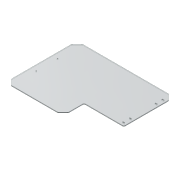
# Autodesk Inventor part: Clear Front Door 2
Saved by Autodesk Inventor 2015 (Build 190159000, 159)
## iProperties
Created: 2018-04-14
Part Number: Clear Front Door 2
Material: Glass
Document SubType Name: Modeling
Designer: Ghassan Yusuf
Density: 2.18 g/cm^3
Appearance: Clear
Author: Ghassan Yusuf
Autodesk Inventor part; units mm, degrees
ref_plane "YZ Plane" through (0, 0, 0) normal (1, 0, 0) x (0, 1, 0)
ref_plane "XZ Plane" through (0, 0, 0) normal (0, 1, 0) x (-1, 0, 0)
ref_plane "XY Plane" through (0, 0, 0) normal (0, 0, 1) x (1, 0, 0)
sketch "TFT LCD Touch Screen" plane through (0, 0, 0) normal (0, 0, 1) x (1, 0, 0)
  line L0 (-55, 32.5) -> (55, 32.5)
  line L1 (55, 32.5) -> (55, -32.5)
  line L2 (55, -32.5) -> (-55, -32.5)
  line L3 (-55, -32.5) -> (-55, 32.5)
  circle A0 centre (-51, 28.5) radius 1.5
  circle A1 centre (-51, -28.5) radius 1.5
  circle A2 centre (51, -28.5) radius 1.5
  circle A3 centre (51, 28.5) radius 1.5
  line L4 (-40, 29) -> (40, 29)
  line L5 (40, 29) -> (40, -29)
  line L6 (40, -29) -> (-40, -29)
  line L7 (-40, -29) -> (-40, 29)
  point P0 (0.75, 3.075)
  point P1 (0, 32.5)
  point P2 (55, 0)
  point P3 (0, 29)
  point P4 (-40, 0)
  dimension "d9" = 110
  dimension "d10" = 65
  dimension "d11" = 3
  dimension "d12" = 57
  dimension "d13" = 102
  dimension "d14" = 4
  dimension "d15" = 4
  dimension "d16" = 80
  dimension "d17" = 58
  measures "d9" distance of L1.end L2.end
  measures "d10" distance of L0.end L1.end
  measures "d11" diameter of A0
  measures "d12" distance of A0.centre A1.centre
  measures "d13" distance of A3.centre A0.centre
  measures "d14" distance from line of L0 A3.centre
  measures "d15" distance from line of L3 A0.centre
  measures "d16" distance of L5.end L6.end
  measures "d17" distance of L4.end L5.end
sketch "Hinges Screw Holes" plane through (0, 0, 0) normal (0, 0, 1) x (1, 0, 0)
  arc A0 (172, 94.429) -> (172, 97.929) centre (172, 96.179) ccw
  arc A1 (172, 68.929) -> (172, 72.429) centre (172, 70.679) ccw
  arc A2 (172, -27.2) -> (172, -23.7) centre (172, -25.45) ccw
  arc A3 (172, -52.7) -> (172, -49.2) centre (172, -50.95) ccw
  arc A4 (167, 97.929) -> (167, 94.429) centre (167, 96.179) ccw
  arc A5 (167, 72.429) -> (167, 68.929) centre (167, 70.679) ccw
  arc A6 (167, -23.7) -> (167, -27.2) centre (167, -25.45) ccw
  arc A7 (167, -49.2) -> (167, -52.7) centre (167, -50.95) ccw
  line L0 (167, 97.929) -> (172, 97.929)
  line L1 (167, 94.429) -> (172, 94.429)
  line L2 (167, 72.429) -> (172, 72.429)
  line L3 (167, 68.929) -> (172, 68.929)
  line L4 (167, -23.7) -> (172, -23.7)
  line L5 (167, -27.2) -> (172, -27.2)
  line L6 (167, -49.2) -> (172, -49.2)
  line L7 (167, -52.7) -> (172, -52.7)
  point P0 (169.5, 0)
  point P1 (0, -7.5)
  dimension "d47" = 3.5
  dimension "d48" = 3.5
  dimension "d50" = 25.5
  dimension "d51" = 3.5
  dimension "d52" = 3.5
  dimension "d53" = 25.5
  dimension "d58" = 3.5
  dimension "d59" = 3.5
  dimension "d60" = 25.5
  dimension "d61" = 3.5
  dimension "d62" = 3.5
  dimension "d63" = 25.5
  dimension "d65" = 5
  dimension "d70" = 78.179
  dimension "d71" = 17.95
  measures "d47" diameter of A0
  measures "d48" diameter of A1
  measures "d50" distance of A1.centre A0.centre
  measures "d51" diameter of A2
  measures "d52" diameter of A3
  measures "d53" distance of A3.centre A2.centre
  measures "d58" diameter of A4
  measures "d59" diameter of A5
  measures "d60" distance of A5.centre A4.centre
  measures "d61" diameter of A6
  measures "d62" diameter of A7
  measures "d63" distance of A7.centre A6.centre
  measures "d65" distance of A0.centre A4.centre
  measures "d70" vertical distance of point (0, -7.5) A1.centre
  measures "d71" vertical distance of A2.centre point (0, -7.5)
sketch "Door Shape" plane through (0, 0, 0) normal (0, 0, 1) x (1, 0, 0)
  line L0 (182, -55.7) -> (182, 113)
  line L1 (182, 113) -> (162, 133)
  line L2 (162, 133) -> (-162, 133)
  line L3 (-162, 133) -> (-182, 113)
  line L4 (-182, 113) -> (-182, -114)
  line L5 (-182, -114) -> (-162, -134)
  line L6 (-162, -134) -> (13.05, -134)
  line L7 (13.05, -134) -> (33.05, -114)
  line L8 (33.05, -114) -> (33.05, -55.7)
  line L9 (33.05, -55.7) -> (182, -55.7)
  line L10 (-161.8343, 132.6) -> (161.8343, 132.6)
  line L11 (161.8343, 132.6) -> (181.6, 112.8343)
  line L12 (181.6, 112.8343) -> (181.6, -55.3)
  line L13 (181.6, -55.3) -> (32.65, -55.3)
  line L14 (32.65, -55.3) -> (32.65, -113.8343)
  line L15 (32.65, -113.8343) -> (12.8843, -133.6)
  line L16 (12.8843, -133.6) -> (-161.8343, -133.6)
  line L17 (-161.8343, -133.6) -> (-181.6, -113.8343)
  line L18 (-181.6, -113.8343) -> (-181.6, 112.8343)
  line L19 (-181.6, 112.8343) -> (-161.8343, 132.6)
  line L20 (12.8843, -133.6) -> (181.6, -133.6)
  line L21 (181.6, -133.6) -> (181.6, -55.3)
  point P0 (-8.285, -11.54)
  dimension "d79" = 0.4
  measures "d79" distance between parallel lines of L2 L10
sketch "Sketch1" plane through (0, 0, 0) normal (0, 0, 1) x (1, 0, 0)
  line L0 (-182, 133.5) -> (182, 133.5)
  line L1 (182, 133.5) -> (182, -133.5)
  line L2 (182, -133.5) -> (-182, -133.5)
  line L3 (-182, -133.5) -> (-182, 133.5)
  line L4 (181.5, 133) -> (-181.5, 133)
  line L5 (-181.5, 133) -> (-181.5, -133)
  line L6 (-181.5, -133) -> (181.5, -133)
  line L7 (181.5, -133) -> (181.5, 133)
  point P0 (0, 0)
  point P1 (0, 133.5)
  point P2 (-181.5, 0)
  dimension "d0" = 364
  dimension "d1" = 267
  dimension "d4" = 0.5
  constraints: 16 end point, 4 parallel, 2 midpoint, 2 perpendicular, 1 horizontal, 1 horizontal alignment, 1 vertical alignment, 3 other
  measures "d0" distance of L1.end L2.end
  measures "d1" distance of L0.end L1.end
  measures "d4" distance between parallel lines of L0 L4
extrude "Extrusion1" add sketch "Sketch1" along normal blind 2.8 contours L7 L6 L5 L4
chamfer "Chamfer1" distance 20 angle 45 4 edges at (-181.5, -133, 1.4) (-181.5, 133, 1.4) (181.5, -133, 1.4) (181.5, 133, 1.4)
fillet "Fillet1" radius 5 8 edges at (-161.5, -133, 1.4) (161.5, -133, 1.4) (181.5, -113, 1.4) (181.5, 113, 1.4) (161.5, 133, 1.4) (-161.5, 133, 1.4) (-181.5, 113, 1.4) (-181.5, -113, 1.4)
sketch "Sketch6" plane through (0, 0, 2.8) normal (0, 0, 1) x (1, 0, 0)
  line L0 (181.5, -110.9289) -> (181.5, 110.9289) projected
  arc A0 (172, 101.929) -> (172, 105.429) centre (172, 103.679) ccw
  arc A1 (172, 76.429) -> (172, 79.929) centre (172, 78.179) ccw
  arc A2 (172, -19.7) -> (172, -16.2) centre (172, -17.95) ccw
  arc A3 (172, -45.2) -> (172, -41.7) centre (172, -43.45) ccw
  arc A4 (167, 105.429) -> (167, 101.929) centre (167, 103.679) ccw
  arc A5 (167, 79.929) -> (167, 76.429) centre (167, 78.179) ccw
  arc A6 (167, -16.2) -> (167, -19.7) centre (167, -17.95) ccw
  arc A7 (167, -41.7) -> (167, -45.2) centre (167, -43.45) ccw
  line L1 (167, 105.429) -> (172, 105.429)
  line L2 (167, 101.929) -> (172, 101.929)
  line L3 (167, 79.929) -> (172, 79.929)
  line L4 (167, 76.429) -> (172, 76.429)
  line L5 (167, -16.2) -> (172, -16.2)
  line L6 (167, -19.7) -> (172, -19.7)
  line L7 (167, -41.7) -> (172, -41.7)
  line L8 (167, -45.2) -> (172, -45.2)
  point P0 (0, 0)
  dimension "d68" = 9.5
  dimension "d69" = 9.5
  dimension "d72" = 78.179
extrude "Extrusion5" cut sketch "Sketch6" against normal blind 10
sketch "Sketch7" plane through (0, 0, 2.8) normal (0, 0, 1) x (1, 0, 0)
  circle A0 centre (-161.5, 40) radius 1.75
  circle A1 centre (-161.5, -40) radius 1.75
  line L0 (-181.5, 110.9289) -> (-181.5, -110.9289) projected
  point P0 (0, 0)
  dimension "d73" = 3.5
  dimension "d74" = 80
  dimension "d75" = 40
  dimension "d76" = 20
  constraints: 2 centre point, 1 equal radius, 1 vertical alignment
  measures "d73" diameter of A0
  measures "d74" distance of A1.centre A0.centre
  measures "d75" vertical distance of point (0, 0) A0.centre
  measures "d76" distance from line of L0 A0.centre
extrude "Extrusion6" cut sketch "Sketch7" against normal blind 18.5
sketch "Sketch8" plane through (0, 0, 2.8) normal (0, 0, 1) x (1, 0, 0)
  line L0 (-181.5, 110.9289) -> (-181.5, -110.9289) projected
  line L1 (159.4289, 133) -> (-159.4289, 133) projected
  line L2 (182, -55.2) -> (182, 113.5)
  line L3 (182, 113.5) -> (162, 133.5)
  line L4 (162, 133.5) -> (-162, 133.5)
  line L5 (-162, 133.5) -> (-182, 113.5)
  line L6 (-182, 113.5) -> (-182, -113.5)
  line L7 (-182, -113.5) -> (-162, -133.5)
  line L8 (-162, -133.5) -> (13.05, -133.5)
  line L9 (13.05, -133.5) -> (33.05, -113.5)
  line L10 (33.05, -113.5) -> (33.05, -55.2)
  line L11 (33.05, -55.2) -> (182, -55.2)
  line L12 (-161.8343, 133.1) -> (161.8343, 133.1)
  line L13 (161.8343, 133.1) -> (181.6, 113.3343)
  line L14 (181.6, 113.3343) -> (181.6, -54.8)
  line L15 (181.6, -54.8) -> (32.65, -54.8)
  line L16 (32.65, -54.8) -> (32.65, -113.3343)
  line L17 (32.65, -113.3343) -> (12.8843, -133.1)
  line L18 (12.8843, -133.1) -> (-161.8343, -133.1)
  line L19 (-161.8343, -133.1) -> (-181.6, -113.3343)
  line L20 (-181.6, -113.3343) -> (-181.6, 113.3343)
  line L21 (-181.6, 113.3343) -> (-161.8343, 133.1)
  line L22 (12.8843, -133.1) -> (181.6, -133.1)
  line L23 (181.6, -133.1) -> (181.6, -54.8)
  point P0 (0, 0)
  point P1 (-182, 0)
  point P2 (-181.5, 0)
  point P3 (0, 133)
  point P4 (0, 133.5)
  constraints: 2 midpoint, 1 horizontal alignment, 1 vertical alignment, 2 other
extrude "Extrusion7" cut sketch "Sketch8" against normal blind 18.5 contours L23 L22 L9 L10 L11 | L11 L10 L9 L22 L17 L16 L15 L23
fillet "Fillet3" radius 5 4 edges at (12.9843, -133, 1.4) (32.65, -113.3343, 1.4) (32.65, -54.8, 1.4) (181.5, -54.8, 1.4)
equation "\"d75\" = 0.5 * d74"
equation "\"d14\" = -0.5 * d12 + 0.5 * d10"
equation "\"d15\" = -0.5 * d13 + 0.5 * d9"
body "Solid1"
